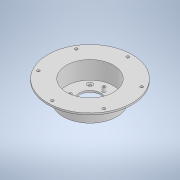
# Autodesk Inventor part: Adapter_motor_planetarygearbox
Saved by Autodesk Inventor 2021 (Build 250183000, 183)
## iProperties
Created: 2020-05-15
Part Number: Adapter_motor_planetarygearbox
Material: Generic
Document SubType Name: Modeling
Designer: avi41
Density: 1 g/cm^3
Appearance: Default
Author: avi41
Autodesk Inventor part; units mm, degrees
ref_plane "YZ Plane" through (0, 0, 0) normal (1, 0, 0) x (0, 1, 0)
ref_plane "XZ Plane" through (0, 0, 0) normal (0, 1, 0) x (-1, 0, 0)
ref_plane "XY Plane" through (0, 0, 0) normal (0, 0, 1) x (1, 0, 0)
sketch "Sketch1" plane through (0, 0, 0) normal (0, 0, 1) x (1, 0, 0)
  line L0 (0, 16.24) -> (0, -16.24) construction
  line L1 (-10, 0) -> (60, 0) construction
  line L2 (50, 11.6) -> (50, 9.6)
  line L3 (50, 9.6) -> (32, 9.6)
  line L4 (28, 11.6) -> (28, -9.6)
  line L5 (28, -9.6) -> (13, -9.6)
  line L6 (13, -9.6) -> (13, -11.6)
  line L7 (13, -11.6) -> (32, -11.6)
  line L8 (32, -11.6) -> (32, 9.6)
  line L9 (28, 11.6) -> (50, 11.6)
  point P0 (0, 0)
  dimension "d0" = 2
  dimension "d1" = 2
  dimension "d4" = 50
  dimension "d7" = 13
  dimension "d11" = 19.2
  dimension "d35" = 32
  dimension "d36" = 4
  dimension "d37" = 21.2
  constraints: 16 end point, 6 perpendicular, 1 other
  measures "d0" distance of L2.start L2.end
  measures "d1" distance of L5.end L6.end
  measures "d4" distance between parallel lines of L0 L2
  measures "d7" distance between parallel lines of L0 L6
  measures "d11" distance between parallel lines of L5 L3
  measures "d35" distance between parallel lines of L0 L8
  measures "d36" distance between parallel lines of L4 L8
  measures "d37" distance between parallel lines of L7 L3
revolve "Revolution1" add sketch "Sketch1" angle 360 about axis through (0, 0, 0) along (0, -1, 0)
sketch "Sketch2" plane through (0, -9.6, 0) normal (0, -1, 0) x (1, 0, 0)
  line L0 (0, 70) -> (0, -70) construction
  line L1 (-70, 0) -> (70, 0) construction
  circle A0 centre (0, 0) radius 13 construction
  circle A1 centre (0, 0) radius 32 construction
  line L2 (15.5, -15.5) -> (-15.5, -15.5) construction
  line L3 (-15.5, -15.5) -> (-15.5, 15.5) construction
  line L4 (-15.5, 15.5) -> (15.5, 15.5) construction
  line L5 (15.5, 15.5) -> (15.5, -15.5) construction
  dimension "d14" = 31
  dimension "d15" = 31
  constraints: 8 end point, 4 coincident, 2 parallel, 1 horizontal, 1 perpendicular, 2 other
  measures "d14" distance of L2.start L2.end
  measures "d15" distance of L2.end L3.end
hole "Hole1" at (15.5, -9.6, -15.5) at (-15.5, -9.6, -15.5) at (-15.5, -9.6, 15.5) at (15.5, -9.6, 15.5) direction (0, -1, 0) diameter 3.4 end through all countersink diameter 6.3 countersink angle 90 clearance for "Flat Head Machine Screw" size "M3" standard "Ansi Metric M Profile"
sketch "Sketch3" plane through (0, 11.6, 0) normal (0, 1, 0) x (1, 0, 0)
  line L0 (0, 70) -> (0, -70) construction
  line L1 (70, 0) -> (-70, 0) construction
  circle A0 centre (0, 0) radius 45 construction
  point P0 (0, 45)
  point P1 (-38.9711, 22.5)
  point P2 (-38.9711, -22.5)
  point P3 (0, -45)
  point P4 (38.9711, -22.5)
  point P5 (38.9711, 22.5)
  dimension "d23" = 90
  dimension "d26" = 360
  constraints: 1 coincident, 1 point on line, 1 vertical alignment, 9 other
hole "Hole2" at (0, 11.6, -45) at (-38.9711, 11.6, -22.5) at (-38.9711, 11.6, 22.5) at (0, 11.6, 45) at (38.9711, 11.6, 22.5) at (38.9711, 11.6, -22.5) direction (0, -1, 0) diameter 3.4 depth 2 tip angle 118 clearance for "Flat Head Machine Screw" size "M3" standard "Ansi Metric M Profile"
fillet "Fillet1" radius 5 1 edges at (-32, 9.6, 0)
sketch "Sketch4" plane through (0, -9.6, 0) normal (0, 1, 0) x (1, 0, 0)
  line L0 (0, 70) -> (0, -70) construction
  line L1 (-70, 0) -> (70, 0) construction
  circle A0 centre (0, 16.6) radius 2
  circle A1 centre (12.5, -11) radius 2
  circle A2 centre (-12.5, -11) radius 2
  point P0 (0, 0)
  dimension "d39" = 4
  dimension "d54" = 16.6
  dimension "d55" = 4
  dimension "d56" = 25
  dimension "d57" = 11
  constraints: 3 centre point, 1 point on line, 1 other
  measures "d39" diameter of A0
  measures "d54" distance from line of A0.centre L1
  measures "d55" diameter of A1
  measures "d56" distance of A1.centre A2.centre
  measures "d57" distance from line of L1 A1.centre
extrude "Extrusion1" add sketch "Sketch4" along normal blind 4.75
sketch "Sketch5" plane through (0, -4.85, -16.6) normal (0, 1, 0) x (1, 0, 0)
  circle A0 centre (0, 0) radius 2 construction
  circle A1 centre (-12.5, -27.6) radius 2 construction
  circle A2 centre (12.5, -27.6) radius 2 construction
  circle A3 centre (12.5, -27.6) radius 2 construction
  point P0 (0, -16.6)
  constraints: 3 coincident
hole "Hole3" at (0, -4.85, -16.6) at (-12.5, -4.85, 11) at (12.5, -4.85, 11) direction (0, -1, 0) diameter 1.567 depth 6.3 tip angle 118 thread size "M2x0.4" class "6H" standard "ANSI Metric M Profile"
equation "\"d55\" = d39"
body "Solid1"
